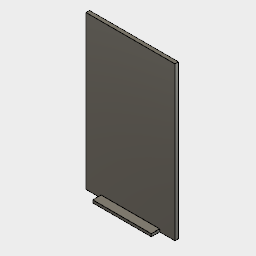
Separator v2 (Autodesk Fusion 360 design; units mm, degrees)
Autodesk Fusion 360 part; units mm, degrees
sketch "Sketch1" plane through (0, 0, 0) normal (0, 1, 0) x (1, 0, 0)
  line L0 (0, 0) -> (31.94, 0)
  line L1 (31.94, 0) -> (31.94, 1.3)
  line L2 (31.94, 1.3) -> (0, 1.3)
  line L3 (0, 1.3) -> (0, 0)
  dimension "d13" = 1.3
  measures "d13" distance of L0.end L1.end
extrude "Extrude1" add sketch "Sketch1" along normal blind 55
sketch "Sketch3" plane through (0, 0, 0) normal (0, -1, 0) x (1, 0, 0)
  line L0 (0, 0) -> (0, -1.3)
  line L1 (0, -1.3) -> (31.94, -1.3)
  line L2 (31.94, -1.3) -> (31.94, 0)
  line L3 (31.94, 0) -> (0, 0)
  line L4 (5.44, 0) -> (26.5, 0)
  line L5 (26.5, 0) -> (26.5, 3)
  line L6 (26.5, 3) -> (5.44, 3)
  line L7 (5.44, 3) -> (5.44, 0)
extrude "Extrude2" add sketch "Sketch3" against normal blind 1 contours L3 L4 L5 L6 L7
